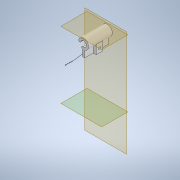
# Autodesk Inventor part: prototype_11(topOnly)
Saved by Autodesk Inventor 2022 (Build 260153000, 153)
## iProperties
Created: 2022-06-15
Part Number: prototype_11(topOnly)
Material: Generic
Document SubType Name: Modeling
Designer: tecware
Density: 1 g/cm^3
Appearance: Default
Author: tecware
## iProperties of the stored document prototype_8_1_3DPrint.ipt
Created: 2022-06-16
Part Number: prototype_8_1_3DPrint
Material: Generic
Document SubType Name: Modeling
Designer: tecware
Density: 1 g/cm^3
Appearance: Default
Author: tecware
Autodesk Inventor part; units mm, degrees
ref_plane "YZ Plane" through (0, 0, 0) normal (1, 0, 0) x (0, 1, 0)
sketch "Sketch1" plane through (0, 0, 0) normal (0, 1, 0) x (-1, 0, 0)
  line L0 (11, -16) -> (-11, -16)
  line L1 (-11, -16) -> (-11, 16)
  line L2 (-11, 16) -> (11, 16)
  line L3 (11, 16) -> (11, -16)
  line L4 (11, -16) -> (-11, 16) construction
  line L5 (-11, -16) -> (11, 16) construction
  circle A0 centre (-2, 6.5) radius 4.8
  line L6 (-2, 6.5) -> (-2, -6.5)
  circle A1 centre (-2, -6.5) radius 4.8
  line L7 (-2, 11.3) -> (-11, 11.3)
  line L8 (-2, 1.7) -> (-11, 1.7)
  line L9 (-2, -1.7) -> (-11, -1.7)
  line L10 (-2, -11.3) -> (-11, -11.3)
  point P0 (0, 0)
  point P1 (-2, 0)
  dimension "d0" = 22
  dimension "d1" = 32
  dimension "d2" = 9.6
  dimension "d3" = 13
  dimension "d4" = 9.6
  constraints: 22 end point, 6 point on line, 4 point on circle, 3 midpoint, 2 centre point, 2 perpendicular, 1 coincident, 1 horizontal, 1 vertical
  measures "d0" distance of L1.end L2.end
  measures "d1" distance of L0.end L1.end
  measures "d2" diameter of A0
  measures "d3" distance of L6.start L6.end
  measures "d4" diameter of A1
extrude "Extrusion1" add sketch "Sketch1" along normal blind 2 contours L0 L1 L10 A1 L6 A0 L7 L2 L3 | L1 L8 L6 L9
sketch "Sketch2" plane through (0, 0, 0) normal (0, -1, 0) x (1, 0, 0)
  line L0 (-11, 16) -> (11, 16) projected
  line L1 (11, 16) -> (-11, 16)
  line L2 (-11, -16) -> (-11, 16) projected
  line L3 (-11, 16) -> (-11, -16)
  line L4 (11, -16) -> (-11, -16) projected
  line L5 (-11, -16) -> (11, -16)
  line L6 (11, -16) -> (11, -14)
  line L7 (11, -11.3) -> (11, -16) projected
  line L8 (11, -14) -> (-5, -14)
  line L9 (-5, -14) -> (-5, 14)
  line L10 (-5, 14) -> (11, 14)
  line L11 (11, 16) -> (11, 11.3) projected
  point P0 (0, 0)
  dimension "d7" = 2
  dimension "d8" = 16
  dimension "d9" = 28
  constraints: 14 end point, 2 point on line
  measures "d7" distance of L4.start L6.end
  measures "d8" distance of L6.end L8.end
  measures "d9" distance of L8.end L9.end
extrude "Extrusion2" add sketch "Sketch2" along normal blind 2.75
sketch "Sketch3" plane through (-11, 2, -16) normal (-1, 0, 0) x (0, 0, 1)
  line L0 (0, 0) -> (0, -4.75) projected
  line L1 (0, -4.75) -> (32, -4.75)
  line L2 (32, -4.75) -> (32, 49.75)
  line L3 (32, 49.75) -> (0, 49.75)
  line L4 (0, 49.75) -> (0, -4.75)
  point P0 (16, -2)
  dimension "d12" = 54.5
  constraints: 8 end point
  measures "d12" distance of L2.end L1.end
extrude "Extrusion3" add sketch "Sketch3" along normal blind 3
sketch "Sketch4" plane through (0, -2.75, 0) normal (0, -1, 0) x (1, 0, 0)
  line L0 (11, 16) -> (11, 11.3) projected
  line L1 (11, 16) -> (-39, 16)
  line L2 (-39, 16) -> (-39, -16)
  line L3 (-39, -16) -> (11, -16)
  line L4 (11, -16) -> (11, 16)
  point P0 (0, 0)
  dimension "d15" = 50
  constraints: 8 end point
  measures "d15" distance of L3.end L2.end
extrude "Extrusion4" add sketch "Sketch4" along normal blind 2
sketch "Sketch5" plane through (-5, 0, 14) normal (1, 0, 0) x (0, 0, -1)
  line L0 (0, 0) -> (0, -2.75) projected
  line L1 (30, -2.75) -> (-2, -2.75) projected
  line L2 (0, 0) -> (2.9896, 0)
  line L3 (2.9896, 0) -> (2.9896, -2.75)
  line L4 (2.9896, -2.75) -> (0, -2.5)
  line L5 (0, -2.5) -> (0, 0)
  point P0 (14, 0)
  dimension "d18" = 3
  constraints: 8 end point, 1 point on line
  measures "d18" distance of L3.end L4.end
extrude "Extrusion5" cut sketch "Sketch5" against normal up to surface (9 mm away)
sketch "Sketch6" plane through (11, 0, 1.7) normal (1, 0, 0) x (0, 0, -1)
  line L0 (0, 0) -> (0, 2) projected
  line L1 (3.4, 0) -> (3.4, 2) projected
  line L2 (0, 1) -> (3.4, 1)
  line L3 (3.4, 1) -> (3.4, 2)
  line L4 (3.4, 2) -> (0, 2)
  line L5 (0, 2) -> (0, 1)
  point P0 (1.7, 0)
  constraints: 8 end point, 1 midpoint
extrude "Extrusion6" cut sketch "Sketch6" against normal blind 2.2
sketch "Sketch8" plane through (-14, 2, -16) normal (-1, 0, 0) x (0, 0, 1)
  circle A0 centre (24.6, 39.75) radius 2.75
  circle A1 centre (24.6, 39.75) radius 1.4
  line L0 (4, 47.25) -> (28, 47.25) construction
  line L1 (28, 47.25) -> (28, -1.75) construction
  line L2 (28, -1.75) -> (4, -1.75) construction
  line L3 (4, -1.75) -> (4, 47.25) construction
  circle A2 centre (7.4, 5.75) radius 2.75
  circle A3 centre (7.4, 5.75) radius 1.4
  line L4 (4, 47.25) -> (28, -1.75) construction
  line L5 (32, -4.75) -> (32, -6.75) construction
  line L6 (32, 49.75) -> (0, 49.75) construction
  line L7 (0, -4.75) -> (32, 49.75) construction
  point P0 (16, -2)
  point P1 (16, 22.75)
  point P2 (16, 22.5)
  dimension "d24" = 5.5
  dimension "d25" = 2.8
  dimension "d26" = 24
  dimension "d27" = 49
  dimension "d28" = 3.4
  dimension "d29" = 7.5
  dimension "d30" = 5.5
  dimension "d31" = 2.8
  dimension "d32" = 3.4
  dimension "d33" = 7.5
  constraints: 12 end point, 4 centre point, 2 coincident, 2 midpoint
  measures "d24" diameter of A0
  measures "d25" diameter of A1
  measures "d26" distance of L1.end L2.end
  measures "d27" distance of L0.end L1.end
  measures "d28" distance from line of L1 A0.centre
  measures "d29" distance from line of L0 A0.centre
  measures "d30" diameter of A2
  measures "d31" diameter of A3
  measures "d32" distance from line of L3 A3.centre
  measures "d33" distance from line of L2 A3.centre
extrude "Extrusion7" add sketch "Sketch8" along normal blind 7
sketch "Sketch9" plane through (0, 0, 0) normal (0, 0, 1) x (1, 0, 0)
  line L0 (-14, -2.75) -> (-14, 51.75) projected
  line L1 (-12.5, 56.75) -> (-12.5, 54.25) construction
  line L2 (-12.25, 56.75) -> (-12.25, 54.25)
  line L3 (-12.25, 54.25) -> (-12.75, 54.25)
  line L4 (-12.75, 54.25) -> (-12.75, 56.75)
  line L5 (-12.75, 56.75) -> (-12.25, 54.25) construction
  line L6 (-12.25, 56.75) -> (-12.75, 54.25) construction
  circle A0 centre (-12.5, 63.45) radius 6.7
  line L7 (-12.5, 63.45) -> (-12.5, 56.75) construction
  line L8 (-12.25, 56.75) -> (-12.25, 59.7585)
  line L9 (-12.75, 59.7585) -> (-12.75, 56.75)
  line L10 (-12.25, 59.7585) -> (-12.25, 70.1453)
  line L11 (-12.25, 70.1453) -> (-12.75, 70.1453)
  line L12 (-12.75, 70.1453) -> (-12.75, 59.7585)
  line L13 (-12.5, 63.45) -> (-5.8, 63.45) construction
  line L14 (-12.5, 63.45) -> (-5.8, 63.45) construction
  line L15 (-11, 51.75) -> (-14, 51.75) projected
  line L16 (-14, 51.75) -> (-11, 51.75)
  line L17 (-11, 51.75) -> (-11, 56.75)
  line L18 (-11, 56.75) -> (-14, 56.75)
  line L19 (-14, 56.75) -> (-14, 51.75)
  line L20 (-14, 56.75) -> (-11, 56.75)
  line L21 (-11, 56.75) -> (-11, 56.9201)
  line L22 (-11, 56.9201) -> (-14, 56.9201)
  line L23 (-14, 56.9201) -> (-14, 56.75)
  line L24 (-12.5, 63.45) -> (-5.8, 63.45) construction
  line L25 (-12.5, 63.45) -> (-5.8, 63.45) construction
  line L26 (-12.5, 63.45) -> (-5.8, 63.45) construction
  circle A1 centre (-12.5, 63.45) radius 3.7
  line L27 (-14, 56.9201) -> (-13.3284, 59.8439)
  line L28 (-12.5, 63.45) -> (-5.8, 63.45) construction
  circle A2 centre (-13.6642, 58.382) radius 1.5
  line L29 (-12.5, 63.45) -> (-7.7359, 63.45) construction
  line L30 (-19.0299, 64.9503) -> (-16.106, 64.2785)
  circle A3 centre (-17.5679, 64.6144) radius 1.5
  point P0 (0, 0)
  point P1 (-12.5, 55.5)
  point P2 (-12.75, 56.7547)
  point P3 (-12.25, 56.7547)
  point P4 (-19.2, 63.45)
  point P5 (-17.2376, 68.1876)
  dimension "d47" = 0.5
  dimension "d50" = 5
  dimension "d128" = 7.4
  dimension "d130" = 13.4
  constraints: 58 end point, 8 point on circle, 7 horizontal, 5 midpoint, 2 centre point, 1 coincident, 1 point on line, 6 other
  measures "d47" distance of L3.start L3.end
  measures "d50" distance of L17.end L16.end
  measures "d128" diameter of A1
  measures "d130" diameter of A0
extrude "Extrusion8" add sketch "Sketch9" along normal mid plane 32 contours L18 L17 L15 L19 L4 L3 L2 | L18 A0 L8 | L8 A0 L21 L18 | L2 L3 L4 L18 | L8 L22 A0 | A0 L9 L22 L8 | L18 L9 A0 | L22 L8 A2 A1 L10 A0 | L22 L9 A2 L8 | L9 L18 L23 A0 | A0 A2 L22 L9 | A2 L9 L8 | L8 A2 | L22 A2 L9 | L27 A2 L9 L22 | A2 L27 | L22 A2 | L11 A0 | L10 A1 L12 L11 | A2 L9 A1 L8 | A3 L30 | A0 L12 A1 A3 | L30 A3 | A1 L9 A2
sketch "Sketch10" plane through (-11, 2, 16) normal (0, 0, 1) x (1, 0, 0)
  line L0 (-1.25, 52.25) -> (-1.25, 37.25)
  line L1 (-1.25, 37.25) -> (-1.75, 37.25)
  line L2 (-1.75, 37.25) -> (-1.75, 52.25)
  arc A0 (-2.2836, 58.0388) -> (-4.9111, 62.2338) centre (-1.5, 61.45) ccw projected
  line L3 (-1.75, 37.25) -> (19.102, 37.25) construction
  arc A1 (-2.2836, 58.0388) -> (-4.9111, 62.2338) centre (-1.5, 61.45) ccw projected
  line L4 (-1.25, 37.25) -> (19.602, 37.25) construction
  point P0 (11, -2)
  point P1 (-3.9749, 63.9249)
  point P2 (-1.75, 57.9589)
  point P3 (-1.25, 57.9589)
  point P4 (0.9749, 63.9249)
  point P5 (-5, 61.45)
  dimension "d51" = 15
  constraints: 10 end point, 2 horizontal
  measures "d51" distance of L0.start L0.end
extrude "Extrusion9" [suppressed]
sketch "Sketch11" plane through (0, 0, 0) normal (0, 0, 1) x (1, 0, 0)
  line L0 (-12.5, 63.45) -> (-18.3024, 60.1)
  line L1 (-14, 56.9201) -> (-14, 62.9804)
  circle A0 centre (-12.5, 63.45) radius 6.7
  point P0 (0, 0)
  point P1 (-14, 62.584)
  constraints: 4 end point, 2 coincident, 3 other
extrude "Extrusion10" cut sketch "Sketch11" along normal mid plane 10 contours L1 A0 L0 picked at (-14.4333, 58.9557)
sketch "Sketch13" plane through (0, 2, 0) normal (0, 1, 0) x (1, 0, 0)
  line L0 (-11, 16) -> (-11, -16) projected
  line L1 (-11, 0) -> (-9, 0) construction
  line L2 (-11, 4.5) -> (-7, 4.5)
  line L3 (-7, 4.5) -> (-7, -4.5)
  line L4 (-7, -4.5) -> (-11, -4.5)
  line L5 (-11, -4.5) -> (-11, 4.5)
  line L6 (-11, 4.5) -> (-7, -4.5) construction
  line L7 (-7, 4.5) -> (-11, -4.5) construction
  point P0 (0, 0)
  point P1 (-11, -4.5)
  dimension "d66" = 2
  dimension "d67" = 4
  dimension "d68" = 9
  constraints: 14 end point, 3 midpoint, 3 perpendicular
  measures "d66" distance of L1.start L1.end
  measures "d67" distance of L3.end L4.end
  measures "d68" distance of L2.end L3.end
extrude "Extrusion12" add sketch "Sketch13" along normal up to surface
sketch "Sketch12" plane through (-14, 2, -16) normal (-1, 0, 0) x (0, 0, 1)
  line L0 (0, 54.9201) -> (32, 54.9201) projected
  line L1 (16, 54.9201) -> (16, 50.9201) construction
  circle A0 centre (16, 50.9201) radius 1.7
  point P0 (16, -2)
  dimension "d62" = 4
  dimension "d63" = 3.4
  constraints: 2 end point, 1 centre point, 1 coincident, 1 midpoint
  measures "d62" distance of L1.start L1.end
  measures "d63" diameter of A0
extrude "Extrusion11" cut sketch "Sketch12" against normal through all
sketch "Sketch14" plane through (-7, 2, 4.5) normal (1, 0, 0) x (0, 0, -1)
  circle A0 centre (4.5, 50.9201) radius 2.9
  point P0 (4.5, -2)
  point P1 (4.5, 50.9201)
  dimension "d96" = 5.8
  constraints: 1 centre point, 1 coincident
  measures "d96" diameter of A0
extrude "Extrusion13" [suppressed]
sketch "Sketch15" plane through (-14, 2, -16) normal (-1, 0, 0) x (0, 0, 1)
  line L0 (0, 28.85) -> (6, 28.85) construction
  line L1 (6, 28.85) -> (6, 16.65) construction
  line L2 (6, 16.65) -> (0, 16.65) construction
  line L3 (0, 16.65) -> (0, 28.85) construction
  line L4 (0, -4.75) -> (0, 54.9201) projected
  line L5 (0, 28.85) -> (6, 28.85)
  line L6 (6, 28.85) -> (6, 30.85)
  line L7 (6, 30.85) -> (0, 30.85)
  line L8 (0, 30.85) -> (0, 28.85)
  line L9 (6, 16.65) -> (0, 16.65)
  line L10 (0, 16.65) -> (0, 14.65)
  line L11 (0, 14.65) -> (6, 14.65)
  line L12 (6, 14.65) -> (6, 16.65)
  circle A0 centre (24.6, 39.75) radius 1.4 projected
  circle A1 centre (7.4, 5.75) radius 1.4 projected
  line L13 (24.6, 39.75) -> (7.4, 5.75)
  line L14 (16, 22.75) -> (-10.8534, 22.75) construction
  line L15 (6, 30.85) -> (8, 30.85)
  line L16 (8, 30.85) -> (8, 14.65)
  line L17 (8, 14.65) -> (6, 14.65)
  line L18 (6, 14.65) -> (6, 30.85)
  point P0 (16, -2)
  point P1 (0, 22.75)
  dimension "d78" = 6
  dimension "d79" = 12.2
  dimension "d80" = 2
  dimension "d81" = 2
  dimension "d101" = 2
  constraints: 36 end point, 2 midpoint, 2 parallel, 2 point on line, 1 collinear, 1 perpendicular, 1 other
  measures "d78" distance of L1.end L2.end
  measures "d79" distance of L0.end L1.end
  measures "d80" distance of L6.end L5.end
  measures "d81" distance of L10.end L9.end
  measures "d101" distance of L16.end L17.end
extrude "Extrusion14" add sketch "Sketch15" along normal blind 6 contours L4 L9 L12 L11 | L4 L7 L6 L5
sketch "Sketch20" plane through (-14, 2, -16) normal (-1, 0, 0) x (0, 0, 1)
  line L0 (6, 14.65) -> (6, 16.65) projected
  line L1 (6.0001, 28.8153) -> (6, 16.65) construction
  line L2 (5, 22.75) -> (6, 22.75) construction
  line L3 (5, 24.75) -> (7, 24.75)
  line L4 (7, 24.75) -> (7, 20.75)
  line L5 (7, 20.75) -> (5, 20.75)
  line L6 (5, 20.75) -> (5, 24.75)
  line L7 (5, 24.75) -> (7, 20.75) construction
  line L8 (7, 24.75) -> (5, 20.75) construction
  line L9 (0, 16.65) -> (0, 28.85) projected
  line L10 (0, 22.75) -> (5, 22.75) construction
  point P0 (16, -2)
  dimension "d102" = 1
  dimension "d103" = 2
  dimension "d104" = 4
  dimension "d109" = 5
  constraints: 18 end point, 3 midpoint
  measures "d102" distance of L2.start L2.end
  measures "d103" distance of L4.end L5.end
  measures "d104" distance of L3.end L4.end
  measures "d109" distance of L10.start L10.end
extrude "Extrusion17" add sketch "Sketch20" along normal blind 1
sketch "Sketch21" plane through (-20, 2, -16) normal (-1, 0, 0) x (0, 0, 1)
  line L0 (0, 54.9201) -> (0, 0) projected
  line L1 (6, 16.65) -> (6, 14.65) projected
  line L2 (0, 30.85) -> (6, 30.85)
  line L3 (6, 30.85) -> (6, 14.65)
  line L4 (6, 14.65) -> (0, 14.65)
  line L5 (0, 14.65) -> (0, 30.85)
  line L6 (6, 30.85) -> (0, 30.85) projected
  point P0 (16, -2)
  point P1 (0, 14.65)
  constraints: 8 end point, 1 collinear, 1 point on line
extrude "Extrusion18" add sketch "Sketch21" along normal blind 1
ref_plane "Work Plane1" through (0, -19.75, 0) normal (0, -1, 0) x (1, 0, 0)
sketch "Sketch16" plane through (0, -19.75, 0) normal (0, -1, 0) x (1, 0, 0)
  line L0 (11, -16) -> (11, 16) projected
  line L1 (11, 16) -> (-39, 16) projected
  line L2 (-39, 16) -> (-39, -16) projected
  line L3 (-39, -16) -> (11, -16) projected
  line L4 (-39, -16) -> (11, -16) projected
  line L5 (-14, 16) -> (-39, 16) projected
  line L6 (11, -16) -> (-39, 16) construction
  circle A0 centre (-14, 0) radius 10.4
  circle A1 centre (-14, 0) radius 13.4
  point P0 (0, 0)
  dimension "d85" = 20.8
  dimension "d86" = 26.8
  constraints: 2 centre point, 2 coincident, 2 end point, 1 midpoint
  measures "d85" diameter of A0
  measures "d86" diameter of A1
extrude "Extrusion15" add sketch "Sketch16" along normal blind 40 contours A1
sketch "Sketch17" plane through (0, -4.75, 0) normal (0, -1, 0) x (1, 0, 0)
  line L0 (11, -16) -> (11, 16) projected
  line L1 (11, 16) -> (-39, 16) projected
  line L2 (-39, 16) -> (-39, -16) projected
  line L3 (-39, -16) -> (11, -16) projected
  point P0 (0, 0)
loft "Loft1" add profiles "Sketch17" section 1 edges at (-27.4, -19.75, 0)
sketch "Sketch18" plane through (0, 0, 0) normal (0, 0, 1) x (1, 0, 0)
  line L0 (-3.6, -19.75) -> (-24.4, -19.75) projected
  line L1 (-14, -19.75) -> (-3.6, -30.15)
  line L2 (-3.6, -59.75) -> (-3.6, -19.75) projected
  line L3 (-14, -19.75) -> (0.7078, -19.75) construction
  line L4 (-14, -19.75) -> (-14, -37.459) construction
  point P0 (0, 0)
  dimension "d93" = 45
  constraints: 6 end point, 1 equal length, 1 horizontal, 1 midpoint, 1 point on line
  measures "d93" angle of L1 L3
revolve "Revolution1" add sketch "Sketch18" angle 360 about axis through (-14, -19.75, 0) along (0, -1, 0)
fillet "Fillet1" [suppressed]
ref_plane "Work Plane2" through (0, 70.15, 0) normal (0, 1, 0) x (-1, 0, 0)
sketch "Sketch19" plane through (0, 70.15, 0) normal (0, 1, 0) x (-1, 0, 0)
  line L0 (5.8, -16) -> (5.8, 16) projected
  line L1 (5.8, 0) -> (19.2, 0)
  circle A0 centre (12.5, 0) radius 1
  point P0 (0, 0)
  dimension "d98" = 2
  constraints: 2 end point, 2 midpoint, 1 centre point, 1 coincident
  measures "d98" diameter of A0
extrude "Extrusion16" [suppressed]
sketch "Sketch22" plane through (0, 0, 0) normal (0, 0, 1) x (1, 0, 0)
  line L0 (-27.4, -59.75) -> (-0.6, -59.75) projected
  line L1 (-14, -59.75) -> (-14, -49.75)
  circle A0 centre (-14, -49.75) radius 2.3
  point P0 (0, 0)
  dimension "d111" = 10
  dimension "d112" = 4.6
  constraints: 2 end point, 1 centre point, 1 coincident, 1 midpoint
  measures "d111" distance of L1.start L1.end
  measures "d112" diameter of A0
extrude "Extrusion19" cut sketch "Sketch22" against normal up to surface
fillet "Fillet2" radius 2 4 edges at (4.1432, -12.25, -11.6117) (-32.1432, -12.25, -11.6117) (-32.1432, -12.25, 11.6117) (4.1432, -12.25, 11.6117)
fillet "Fillet3" radius 50 5 edges at (-14, -19.75, 13.4) (-27.4, -19.75, 0) (-14, -19.75, -13.4) (-1.1392, -19.75, 3.7631) (-1.1392, -19.75, -3.7631)
fillet "Fillet4" [suppressed]
chamfer "Chamfer1" distance 1 angle 45 2 edges at (-15, 22.75, -10) (-15, 26.75, -10)
ref_plane "Work Plane3" through (0, 0, -15.9) normal (0, 0, 1) x (1, 0, 0)
sketch "Sketch25" plane through (0, 0, -15.9) normal (0, 0, 1) x (1, 0, 0)
  spline S0 degree 8 poles (-11.7, -49.75) (-11.7, -49.5097) (-11.7287, -49.2698) (-11.7859, -49.0321) (-11.8723, -48.7988) (-11.9888, -48.5725) (-12.137, -48.3567) (-12.3183, -48.1562) (-12.7177, -47.8258) (-12.9335, -47.6839) (-13.1784, -47.5646) (-13.4462, -47.4772) (-13.7287, -47.428) (-14.0168, -47.4199) (-14.3008, -47.4526) (-14.852, -47.5941) (-15.1085, -47.7029) (-15.3387, -47.8407) (-15.5414, -48.0011) (-15.7165, -48.1787) (-15.8642, -48.3688) (-15.9854, -48.5672) (-16.1908, -49.0039) (-16.2689, -49.2473) (-16.3156, -49.4971) (-16.3311, -49.75) (-16.3156, -50.0029) (-16.2689, -50.2527) (-16.1908, -50.4961) (-15.9913, -50.9202) (-15.8793, -51.1063) (-15.7442, -51.285) (-15.5854, -51.4532) (-15.4024, -51.6074) (-15.195, -51.7431) (-14.9639, -51.8552) (-14.4711, -52.0153) (-14.2151, -52.0653) (-13.95, -52.0819) (-13.6839, -52.0629) (-13.4255, -52.009) (-13.1825, -51.9242) (-12.9617, -51.8152) (-12.4907, -51.5162) (-12.2578, -51.3051) (-12.0678, -51.0702) (-11.9188, -50.8193) (-11.8088, -50.5579) (-11.7362, -50.2904) (-11.7, -50.02) (-11.7, -49.75) knots 0 0 0 0 0 0 0 0 0 0.154765 0.154765 0.154765 0.154765 0.154765 0.154765 0.154765 0.286658 0.286658 0.286658 0.286658 0.286658 0.286658 0.286658 0.422821 0.422821 0.422821 0.422821 0.422821 0.422821 0.422821 0.578882 0.578882 0.578882 0.578882 0.578882 0.578882 0.578882 0.706632 0.706632 0.706632 0.706632 0.706632 0.706632 0.706632 0.827549 0.827549 0.827549 0.827549 0.827549 0.827549 0.827549 1 1 1 1 1 1 1 1 1 projected
  line L0 (-27.4, -59.75) -> (-0.6, -59.75) projected
  line L1 (-12.4508, -48.05) -> (-16.2649, -50.1503) construction
  line L2 (-12.0685, -50.9987) -> (-15.8752, -51.0817) construction
  line L3 (-13.9718, -51.0402) -> (-14.0129, -49.1567) construction
  line L4 (-14.3578, -49.1002) -> (-13.757, -50.1913) construction
  circle A0 centre (-14, -49.75) radius 4.3
  point P0 (0, 0)
  dimension "d125" = 8.6
  constraints: 8 end point, 2 midpoint, 2 point on line, 1 centre point, 1 coincident, 5 other
  measures "d125" diameter of A0
extrude "Extrusion21" add sketch "Sketch25" along normal up to surface
sketch "Sketch26" plane through (11, 2, -16) normal (0, 0, -1) x (-1, 0, 0)
  line L0 (5.7835, 45.7367) -> (45.0889, 45.7367)
  point P0 (11, -2)
  constraints: 2 end point
split body "Split1" sketch "Sketch26" result one side removed curves L0 removed pieces at (-13.9348, -47.852, 12.8998)
body "Solid1"
